Autodesk Fusion 360 part; units mm, degrees
(part 7 of 7)
  line L1008 (-19.5, -38.2) -> (-19.5, -32.2)
  line L1009 (-19.5, -32.2) -> (-19.5, -35.3676)
  circle A467 centre (-16.25, -62.1) radius 2.5
  circle A468 centre (-16.25, -62.1) radius 2.5
  line L1010 (34.2, 32.4) -> (59.7, 32.4)
  line L1011 (59.7, 32.4) -> (34.2, 32.4)
  line L1012 (95.9, -24.9) -> (101.9, -24.9)
  line L1013 (101.9, -24.9) -> (95.9, -24.9)
  line L1014 (-6.9778, -6.9) -> (-2, -6.9)
  line L1015 (-2, -6.9) -> (-2, -1.9)
  line L1016 (-2, -1.9) -> (-6.9716, -1.9)
  line L1017 (-6.9716, -1.9) -> (-6.9778, -6.9)
  line L1018 (46.45, -80.6) -> (45.65, -80.6)
  line L1019 (45.65, -80.6) -> (46.45, -80.6)
  line L1020 (107.65, -38.95) -> (107.65, -43.95)
  line L1021 (107.65, -43.95) -> (107.65, -38.95)
  line L1022 (-19.5, -44.7) -> (-19.5, -47.5324)
  line L1023 (-19.5, -47.5324) -> (-19.5, -50.7)
  line L1024 (-19.5, -50.7) -> (-19.5, -44.7)
  circle A469 centre (-16.25, -62.1) radius 0.4
  circle A470 centre (-16.25, -62.1) radius 0.4
  line L1025 (-2, -18.9) -> (-6.9926, -18.9)
  line L1026 (-6.9926, -18.9) -> (-2, -18.9)
  arc A471 (64.7, 8) -> (66.7, 10) centre (64.7, 10) ccw
  arc A472 (64.7, 8) -> (66.7, 10) centre (64.7, 10) ccw
  line L1027 (64.7, 8) -> (29.2, 8)
  line L1028 (29.2, 8) -> (64.7, 8)
  line L1029 (59.7, 32.4) -> (59.7, 30.4)
  line L1030 (59.7, 30.4) -> (59.7, 32.4)
  line L1031 (-6.9926, -18.9) -> (-6.9864, -13.9)
  line L1032 (-6.9864, -13.9) -> (-6.9926, -18.9)
  line L1033 (-19.5, -38.2) -> (-19.5, -35.3676)
  arc A473 (-19.5, -35.3676) -> (-22.3324, -38.2) centre (-16.25, -41.45) ccw
  line L1034 (-22.3324, -38.2) -> (-19.5, -38.2)
  line L1035 (59.7, 30.4) -> (66.7, 30.4)
  line L1036 (66.7, 30.4) -> (59.7, 30.4)
  line L1037 (107.2148, -43.61) -> (107.185, -39.2283)
  arc A474 (107.185, -39.2283) -> (98.0852, -39.29) centre (102.65, -41.45) ccw
  line L1038 (98.0852, -39.29) -> (98.115, -43.6717)
  arc A475 (98.115, -43.6717) -> (105.2701, -45.7671) centre (102.65, -41.45) ccw
  line L1039 (105.2701, -45.7671) -> (105.6552, -46.1523)
  line L1040 (105.6552, -46.1523) -> (107.3523, -44.4552)
  line L1041 (107.3523, -44.4552) -> (106.9671, -44.0701)
  arc A476 (106.9671, -44.0701) -> (107.2148, -43.61) centre (102.65, -41.45) ccw
  circle A477 centre (102.65, -41.45) radius 3.85
  line L1042 (-21.2106, -67.0687) -> (-21.5816, -73.1909)
  line L1043 (-21.5816, -73.1909) -> (-21.2106, -67.0687)
  line L1044 (101.9, -25.9) -> (95.9, -25.9)
  line L1045 (95.9, -25.9) -> (101.9, -25.9)
  line L1046 (101.9, -24.9) -> (101.9, -25.9)
  line L1047 (101.9, -25.9) -> (101.9, -24.9)
  arc A478 (-22.3324, -44.7) -> (-19.5, -47.5324) centre (-16.25, -41.45) ccw
  arc A479 (-22.3324, -44.7) -> (-19.5, -47.5324) centre (-16.25, -41.45) ccw
  line L1048 (-19.5, -44.7) -> (-22.3324, -44.7)
  arc A480 (-22.3324, -44.7) -> (-19.5, -47.5324) centre (-16.25, -41.45) ccw
  line L1049 (-19.5, -47.5324) -> (-19.5, -44.7)
  line L1050 (45.65, -79.6) -> (46.45, -79.6)
  line L1051 (46.45, -79.6) -> (45.65, -79.6)
  circle A481 centre (102.65, -41.45) radius 3.85
  circle A482 centre (102.65, -41.45) radius 3.85
  line L1052 (-7.5, -83.1) -> (-12.5, -83.1)
  line L1053 (-12.5, -83.1) -> (-7.5, -83.1)
  line L1054 (114.8523, -45.9448) -> (113.1552, -44.2477)
  line L1055 (113.1552, -44.2477) -> (114.8523, -45.9448)
  line L1056 (-12.5, -78.1) -> (-7.5, -83.1)
  line L1057 (-7.5, -83.1) -> (-12.5, -78.1)
  line L1058 (-7, 4.1) -> (-7, 2)
  line L1059 (-7, 2) -> (-7, 1.6)
  line L1060 (-7, 1.6) -> (-7, 4.1)
  line L1061 (48.25, -80.6) -> (47.45, -80.6)
  line L1062 (47.45, -80.6) -> (48.25, -80.6)
  line L1063 (114.4671, -46.3299) -> (114.8523, -45.9448)
  line L1064 (114.8523, -45.9448) -> (114.4671, -46.3299)
  line L1065 (-25.5, -38.2) -> (-25.5, -44.7)
  line L1066 (-25.5, -44.7) -> (-25.5, -38.2)
  line L1067 (-4.5, 4.1) -> (-7, 4.1)
  line L1068 (-7, 4.1) -> (-4.5, 4.1)
  line L1069 (112.7701, -44.6329) -> (113.1552, -44.2477)
  line L1070 (113.1552, -44.2477) -> (112.7701, -44.6329)
  line L1071 (-15.3557, -72.8958) -> (-20.5769, -73.1432)
  line L1072 (-20.5769, -73.1432) -> (-15.3557, -72.8958)
  arc A483 (-20.2671, -68.0326) -> (-15.3557, -72.8958) centre (-12.5, -65.1) ccw
  arc A484 (-20.2671, -68.0326) -> (-15.3557, -72.8958) centre (-12.5, -65.1) ccw
  arc A485 (48.25, -80.6) -> (48.25, -79.6) centre (48.25, -80.1) ccw
  arc A486 (48.25, -80.6) -> (48.25, -79.6) centre (48.25, -80.1) ccw
  line L1073 (-22.3324, -44.7) -> (-19.5, -44.7)
  line L1074 (-19.5, -44.7) -> (-25.5, -44.7)
  line L1075 (-25.5, -44.7) -> (-22.3324, -44.7)
  circle A487 centre (-4.5, 1.6) radius 0.4
  circle A488 centre (-4.5, 1.6) radius 0.4
  line L1076 (-10.1676, -38.2) -> (-13, -38.2)
  line L1077 (-13, -38.2) -> (-7, -38.2)
  line L1078 (-7, -38.2) -> (-10.1676, -38.2)
  arc A489 (-6.9678, 1.2) -> (-4.5, -0.9) centre (-4.5, 1.6) ccw
  arc A490 (-7, 1.6) -> (-4.5, -0.9) centre (-4.5, 1.6) ccw
  arc A491 (-7, 1.6) -> (-6.9678, 1.2) centre (-4.5, 1.6) ccw
  arc A492 (47.45, -79.6) -> (46.45, -79.6) centre (46.95, -79.6) ccw
  line L1079 (47.45, -79.6) -> (48.25, -79.6)
  arc A493 (48.25, -80.6) -> (48.25, -79.6) centre (48.25, -80.1) ccw
  line L1080 (48.25, -80.6) -> (47.45, -80.6)
  arc A494 (46.45, -80.6) -> (47.45, -80.6) centre (46.95, -80.6) ccw
  line L1081 (46.45, -80.6) -> (45.65, -80.6)
  arc A495 (45.65, -79.6) -> (45.65, -80.6) centre (45.65, -80.1) ccw
  line L1082 (45.65, -79.6) -> (46.45, -79.6)
  circle A496 centre (46.95, -80.1) radius 2.95
  circle A497 centre (-4.5, 1.6) radius 0.4
  line L1083 (113.1, -39.2591) -> (113.1, -43.6409)
  line L1084 (113.1, -43.6409) -> (113.1, -39.2591)
  line L1085 (122.2, -43.6409) -> (122.2, -39.2591)
  line L1086 (122.2, -39.2591) -> (122.2, -43.6409)
  line L1087 (-4.5, -0.9) -> (-2, -0.9)
  line L1088 (-2, -0.9) -> (-4.5, -0.9)
  line L1089 (13.4164, 23.7) -> (10.7819, 23.7)
  line L1090 (10.7819, 23.7) -> (27.2, 23.7)
  line L1091 (27.2, 23.7) -> (13.4164, 23.7)
  line L1092 (-6.5, -83.1) -> (-12.5, -77.1)
  line L1093 (-12.5, -77.1) -> (-6.5, -83.1)
  arc A498 (-20.617, -81.166) -> (-13.5, -83.0722) centre (-12.5, -65.1) ccw
  arc A499 (-20.617, -81.166) -> (-13.5, -83.0722) centre (-12.5, -65.1) ccw
  arc A500 (112.3409, -38.5) -> (112.3409, -29.4) centre (110.15, -33.95) ccw
  arc A501 (112.3409, -38.5) -> (112.3409, -29.4) centre (110.15, -33.95) ccw
  line L1094 (107.9591, -38.5) -> (112.3409, -38.5)
  line L1095 (112.3409, -38.5) -> (107.9591, -38.5)
  line L1096 (13.4164, 15.7) -> (27.2, 15.7)
  line L1097 (27.2, 15.7) -> (10.7819, 15.7)
  line L1098 (10.7819, 15.7) -> (13.4164, 15.7)
  line L1099 (122.2, -43.6409) -> (122.2, -39.2591)
  arc A502 (122.2, -39.2591) -> (115.0299, -37.1329) centre (117.65, -41.45) ccw
  line L1100 (115.0299, -37.1329) -> (114.6448, -36.7477)
  line L1101 (114.6448, -36.7477) -> (112.9477, -38.4448)
  line L1102 (112.9477, -38.4448) -> (113.3329, -38.8299)
  arc A503 (113.3329, -38.8299) -> (113.1, -39.2591) centre (117.65, -41.45) ccw
  line L1103 (113.1, -39.2591) -> (113.1, -43.6409)
  arc A504 (113.1, -43.6409) -> (122.2, -43.6409) centre (117.65, -41.45) ccw
  circle A505 centre (117.65, -41.45) radius 3.85
  line L1104 (0, 4.1) -> (-2, 4.1)
  line L1105 (-2, 4.1) -> (-4.5, 4.1)
  line L1106 (-4.5, 4.1) -> (0, 4.1)
  line L1107 (-13, -32.2) -> (-19.5, -32.2)
  line L1108 (-19.5, -32.2) -> (-13, -32.2)
  line L1109 (-27.8571, -74.4894) -> (-21.6425, -74.1949)
  line L1110 (-21.6425, -74.1949) -> (-27.8571, -74.4894)
  line L1111 (47.45, -79.6) -> (48.25, -79.6)
  line L1112 (48.25, -79.6) -> (47.45, -79.6)
  line L1113 (-13.5, -74.049) -> (-13.5, -83.0722)
  line L1114 (-13.5, -83.0722) -> (-13.5, -74.049)
  line L1115 (-19.5, -50.7) -> (-13, -50.7)
  line L1116 (-13, -50.7) -> (-19.5, -50.7)
  line L1117 (-23, 22.8505) -> (-23, 4.0495)
  line L1118 (-23, 4.0495) -> (-23, 22.8505)
  arc A506 (-27.8571, -74.4894) -> (-22.0173, -80.3781) centre (-12.5, -65.1) ccw
  line L1119 (-22.0173, -80.3781) -> (-21.6425, -74.1949)
  line L1120 (-21.6425, -74.1949) -> (-27.8571, -74.4894)
  line L1121 (-21.0008, -80.1355) -> (-14.7326, -73.8674)
  line L1122 (-14.7326, -73.8674) -> (-20.6378, -74.1472)
  line L1123 (-20.6378, -74.1472) -> (-21.0008, -80.1355)
  line L1124 (-8.1652, 16.7) -> (8.1652, 16.7)
  line L1125 (8.1652, 16.7) -> (-8.1652, 16.7)
  line L1126 (-20.5769, -73.1432) -> (-15.3557, -72.8958)
  arc A507 (-20.2671, -68.0326) -> (-15.3557, -72.8958) centre (-12.5, -65.1) ccw
  line L1127 (-20.2671, -68.0326) -> (-20.5769, -73.1432)
  line L1128 (118.9, -24.9) -> (119.9, -24.9)
  line L1129 (119.9, -24.9) -> (118.9, -24.9)
  line L1130 (112.3409, -29.4) -> (107.9591, -29.4)
  line L1131 (107.9591, -29.4) -> (112.3409, -29.4)
  line L1132 (112.3409, -44.4) -> (107.9591, -44.4)
  line L1133 (107.9591, -44.4) -> (112.3409, -44.4)
  arc A508 (-8.1652, 16.7) -> (-8.1652, 14.7) centre (-8.1652, 15.7) ccw
  arc A509 (-8.1652, 16.7) -> (-8.1652, 14.7) centre (-8.1652, 15.7) ccw
  line L1134 (-20.5769, -73.1432) -> (-20.2671, -68.0326)
  line L1135 (-20.2671, -68.0326) -> (-20.5769, -73.1432)
  line L1136 (-22, 4.0495) -> (-22, 22.8505)
  line L1137 (-22, 22.8505) -> (-22, 4.0495)
  line L1138 (-12.5, -78.1) -> (-12.5, -83.1)
  line L1139 (-12.5, -83.1) -> (-7.5, -83.1)
  line L1140 (-7.5, -83.1) -> (-12.5, -78.1)
  arc A510 (113.1, -43.6409) -> (122.2, -43.6409) centre (117.65, -41.45) ccw
  arc A511 (113.1, -43.6409) -> (122.2, -43.6409) centre (117.65, -41.45) ccw
  line L1141 (-13, -47.5324) -> (-13, -44.7)
  line L1142 (-13, -44.7) -> (-13, -50.7)
  line L1143 (-13, -50.7) -> (-13, -47.5324)
  line L1144 (-20.6378, -74.1472) -> (-14.7326, -73.8674)
  line L1145 (-14.7326, -73.8674) -> (-20.6378, -74.1472)
  line L1146 (-21.0008, -80.1355) -> (-20.6378, -74.1472)
  line L1147 (-20.6378, -74.1472) -> (-21.0008, -80.1355)
  line L1148 (-20.617, -81.166) -> (-13.5, -74.049)
  line L1149 (-13.5, -74.049) -> (-20.617, -81.166)
  arc A512 (112.7701, -44.6329) -> (112.3409, -44.4) centre (110.15, -48.95) ccw
  arc A513 (112.7701, -44.6329) -> (112.3409, -44.4) centre (110.15, -48.95) ccw
  line L1150 (-14.7326, -73.8674) -> (-21.0008, -80.1355)
  line L1151 (-21.0008, -80.1355) -> (-14.7326, -73.8674)
  arc A514 (-27.8571, -74.4894) -> (-22.0173, -80.3781) centre (-12.5, -65.1) ccw
  arc A515 (-27.8571, -74.4894) -> (-22.0173, -80.3781) centre (-12.5, -65.1) ccw
  arc A516 (122.2, -39.2591) -> (115.0299, -37.1329) centre (117.65, -41.45) ccw
  arc A517 (122.2, -39.2591) -> (115.0299, -37.1329) centre (117.65, -41.45) ccw
  line L1152 (-21.6425, -74.1949) -> (-22.0173, -80.3781)
  line L1153 (-22.0173, -80.3781) -> (-21.6425, -74.1949)
  line L1154 (115.0299, -37.1329) -> (114.6448, -36.7477)
  line L1155 (114.6448, -36.7477) -> (115.0299, -37.1329)
  line L1156 (113.3329, -38.8299) -> (112.9477, -38.4448)
  line L1157 (112.9477, -38.4448) -> (113.3329, -38.8299)
  arc A518 (113.3329, -38.8299) -> (113.1, -39.2591) centre (117.65, -41.45) ccw
  arc A519 (113.3329, -38.8299) -> (113.1, -39.2591) centre (117.65, -41.45) ccw
  arc A520 (47.45, -79.6) -> (46.45, -79.6) centre (46.95, -79.6) ccw
  arc A521 (47.45, -79.6) -> (46.45, -79.6) centre (46.95, -79.6) ccw
  arc A522 (0, 5.7) -> (8.6603, 8.7) centre (0, 19.7) ccw
  line L1158 (0, 5.7) -> (0, 4.1)
  line L1159 (0, 4.1) -> (27.2, 4.1)
  line L1160 (27.2, 4.1) -> (27.2, 8.7)
  line L1161 (27.2, 8.7) -> (8.6603, 8.7)
  circle A523 centre (46.95, -80.1) radius 2.95
  arc A524 (46.4092, -77.2) -> (47.4908, -77.2) centre (46.95, -80.1) ccw
  arc A525 (47.4908, -77.2) -> (46.4092, -77.2) centre (46.95, -80.1) ccw
  line L1162 (27.2, 30.4) -> (34.2, 30.4)
  line L1163 (34.2, 30.4) -> (27.2, 30.4)
  arc A526 (-19.8023, -65.1) -> (-12.5, -72.4023) centre (-12.5, -65.1) ccw
  arc A527 (-19.8023, -65.1) -> (-12.5, -72.4023) centre (-12.5, -65.1) ccw
  line L1164 (-23, 22.8505) -> (-23, 4.0495)
  arc A528 (-22, 4.0495) -> (-23, 4.0495) centre (-22.5, 1.6) ccw
  line L1165 (-22, 4.0495) -> (-22, 22.8505)
  arc A529 (-23, 22.8505) -> (-22, 22.8505) centre (-22.5, 25.3) ccw
  line L1166 (-12.5, -77.1) -> (-12.5, -72.4023)
  line L1167 (-12.5, -72.4023) -> (-12.5, -77.1)
  line L1168 (-12.5, -84.1) -> (-6.5, -84.1)
  line L1169 (-6.5, -84.1) -> (-12.5, -84.1)
  line L1170 (27.2, 15.7) -> (13.4164, 15.7)
  arc A530 (8.6603, 8.7) -> (13.4164, 15.7) centre (0, 19.7) ccw
  line L1171 (8.6603, 8.7) -> (27.2, 8.7)
  line L1172 (27.2, 8.7) -> (27.2, 15.7)
  arc A531 (8.1652, 14.7) -> (8.1652, 16.7) centre (8.1652, 15.7) ccw
  arc A532 (8.1652, 14.7) -> (8.1652, 16.7) centre (8.1652, 15.7) ccw
  arc A533 (-20.617, -81.166) -> (-13.5, -83.0722) centre (-12.5, -65.1) ccw
  line L1173 (-13.5, -83.0722) -> (-13.5, -74.049)
  line L1174 (-13.5, -74.049) -> (-20.617, -81.166)
  line L1175 (-31.5, 4.1) -> (-31.5, 25.3)
  line L1176 (-31.5, 25.3) -> (-31.5, 4.1)
  line L1177 (124.4, -7.9) -> (124.4, -12.9)
  line L1178 (124.4, -12.9) -> (124.4, -7.9)
  line L1179 (119.9, -0.9) -> (119.9, 4.1)
  line L1180 (119.9, 4.1) -> (119.9, -0.9)
  line L1181 (98.4, 4.1) -> (95.9, 4.1)
  line L1182 (95.9, 4.1) -> (98.4, 4.1)
  line L1183 (124.4, -0.9) -> (119.9, -0.9)
  line L1184 (119.9, -0.9) -> (124.4, -0.9)
  arc A534 (102.0652, 14.7) -> (102.0652, 16.7) centre (102.0652, 15.7) ccw
  arc A535 (102.0652, 14.7) -> (102.0652, 16.7) centre (102.0652, 15.7) ccw
  line L1185 (85.7348, 24.7) -> (102.0652, 24.7)
  line L1186 (102.0652, 24.7) -> (85.7348, 24.7)
  line L1187 (102.9, 18.7) -> (84.9, 18.7)
  line L1188 (84.9, 18.7) -> (102.9, 18.7)
  line L1189 (95.9, 4.1) -> (93.9, 4.1)
  line L1190 (93.9, 4.1) -> (95.9, 4.1)
  line L1191 (118.9, 1.6) -> (118.9, 4.1)
  line L1192 (118.9, 4.1) -> (118.9, 1.6)
  arc A536 (83.1181, 15.7) -> (83.1181, 23.7) centre (93.9, 19.7) ccw
  arc A537 (83.1181, 15.7) -> (83.1181, 23.7) centre (93.9, 19.7) ccw
  line L1193 (98.9, 10.7) -> (88.9, 10.7)
  line L1194 (88.9, 10.7) -> (98.9, 10.7)
  line L1195 (107.9, -0.9) -> (107.9, 1.2)
  line L1196 (107.9, 1.2) -> (107.9, -0.9)
  line L1197 (116.9, 4.0495) -> (116.9, 22.8505)
  arc A538 (115.9, 22.8505) -> (116.9, 22.8505) centre (116.4, 25.3) ccw
  line L1198 (115.9, 22.8505) -> (115.9, 4.0495)
  arc A539 (116.9, 4.0495) -> (115.9, 4.0495) centre (116.4, 1.6) ccw
  circle A540 centre (116.4, 25.3) radius 2.5
  arc A541 (116.9, 22.8505) -> (115.9, 22.8505) centre (116.4, 25.3) ccw
  arc A542 (115.9, 22.8505) -> (116.9, 22.8505) centre (116.4, 25.3) ccw
  line L1199 (107.9, 1.2) -> (107.9, -0.9)
  line L1200 (107.9, -0.9) -> (112.9, -0.9)
  line L1201 (112.9, -0.9) -> (112.9, 1.2)
  line L1202 (112.9, 1.2) -> (107.9, 1.2)
  line L1203 (116.4, -0.9) -> (113.9, -0.9)
  line L1204 (113.9, -0.9) -> (116.4, -0.9)
  arc A543 (102.0652, 22.7) -> (102.0652, 24.7) centre (102.0652, 23.7) ccw
  arc A544 (102.0652, 22.7) -> (102.0652, 24.7) centre (102.0652, 23.7) ccw
  line L1205 (113.9, 1.2) -> (113.9, -0.9)
  line L1206 (113.9, -0.9) -> (116.4, -0.9)
  arc A545 (113.9322, 1.2) -> (116.4, -0.9) centre (116.4, 1.6) ccw
  line L1207 (113.9322, 1.2) -> (113.9, 1.2)
  line L1208 (124.4, -0.9) -> (124.4, 4.1)
  line L1209 (124.4, 4.1) -> (119.9, 4.1)
  line L1210 (119.9, 4.1) -> (119.9, -0.9)
  line L1211 (119.9, -0.9) -> (124.4, -0.9)
  circle A546 centre (116.4, 25.3) radius 0.4
  circle A547 centre (116.4, 25.3) radius 0.4
  line L1212 (88.8996, 12.7) -> (98.8996, 12.7)
  line L1213 (98.8996, 12.7) -> (88.8996, 12.7)
  circle A548 centre (110.2363, -20.8316) radius 0.4
  circle A549 centre (110.2363, -20.8316) radius 0.4
  line L1214 (118.9, -24.9) -> (118.9, -25.9)
  line L1215 (118.9, -25.9) -> (124.4, -25.9)
  line L1216 (124.4, -25.9) -> (124.4, -24.9)
  line L1217 (124.4, -24.9) -> (124.4, -19.9)
  line L1218 (124.4, -19.9) -> (119.9, -19.9)
  line L1219 (119.9, -19.9) -> (119.9, -24.9)
  line L1220 (119.9, -24.9) -> (118.9, -24.9)
  arc A550 (116.4, 2) -> (116.3992, 1.2) centre (116.4, 1.6) ccw
  arc A551 (116.3992, 1.2) -> (116.4, 2) centre (116.4, 1.6) ccw
  line L1221 (119.9, -12.9) -> (119.9, -7.9)
  line L1222 (119.9, -7.9) -> (119.9, -12.9)
  line L1223 (98.9004, 26.7) -> (88.8996, 26.7)
  line L1224 (88.8996, 26.7) -> (98.9004, 26.7)
  arc A552 (98.9004, 26.7) -> (98.9, 28.7) centre (98.9, 27.7) ccw
  arc A553 (98.9004, 26.7) -> (98.9, 28.7) centre (98.9, 27.7) ccw
  line L1225 (119.9, -19.9) -> (124.4, -19.9)
  line L1226 (124.4, -19.9) -> (119.9, -19.9)
  line L1227 (116.4, -0.9) -> (118.9, -0.9)
  line L1228 (118.9, -0.9) -> (116.4, -0.9)
  line L1229 (124.4, 4.1) -> (124.4, -0.9)
  line L1230 (124.4, -0.9) -> (124.4, 4.1)
  line L1231 (113.9, -0.9) -> (113.9, 1.2)
  line L1232 (113.9, 1.2) -> (113.9, -0.9)
  line L1233 (100.8678, 1.2) -> (100.8704, -0.9)
  line L1234 (100.8704, -0.9) -> (100.8678, 1.2)
  line L1235 (119.9, -7.9) -> (124.4, -7.9)
  line L1236 (124.4, -7.9) -> (119.9, -7.9)
  line L1237 (116.4, -0.9) -> (118.9, -0.9)
  line L1238 (118.9, -0.9) -> (118.9, 1.6)
  arc A554 (116.4, -0.9) -> (118.9, 1.6) centre (116.4, 1.6) ccw
  line L1239 (100.9, 4.1) -> (98.4, 4.1)
  line L1240 (98.4, 4.1) -> (100.9, 4.1)
  line L1241 (98.4, -0.9) -> (100.8704, -0.9)
  line L1242 (100.8704, -0.9) -> (100.8678, 1.2)
  arc A555 (98.4, -0.9) -> (100.8678, 1.2) centre (98.4, 1.6) ccw
  line L1243 (118.9, 1.6) -> (118.9, -0.9)
  line L1244 (118.9, -0.9) -> (118.9, 1.6)
  arc A556 (98.9, 10.7) -> (98.8996, 12.7) centre (98.9, 11.7) ccw
  arc A557 (98.9, 10.7) -> (98.8996, 12.7) centre (98.9, 11.7) ccw
  circle A558 centre (116.4, 25.3) radius 0.4
  line L1245 (119.9, -7.9) -> (119.9, -12.9)
  line L1246 (119.9, -12.9) -> (124.4, -12.9)
  line L1247 (124.4, -12.9) -> (124.4, -7.9)
  line L1248 (124.4, -7.9) -> (119.9, -7.9)
  line L1249 (112.9, -0.9) -> (107.9, -0.9)
  line L1250 (107.9, -0.9) -> (112.9, -0.9)
  line L1251 (85.7348, 16.7) -> (102.0652, 16.7)
  line L1252 (102.0652, 16.7) -> (85.7348, 16.7)
  circle A559 centre (110.2363, -20.8316) radius 0.4
  line L1253 (102.0652, 14.7) -> (85.7348, 14.7)
  line L1254 (85.7348, 14.7) -> (102.0652, 14.7)
  line L1255 (98.4, -0.9) -> (100.8704, -0.9)
  line L1256 (100.8704, -0.9) -> (98.4, -0.9)
  arc A560 (102.9, 18.7) -> (102.9, 20.7) centre (102.9, 19.7) ccw
  arc A561 (102.9, 18.7) -> (102.9, 20.7) centre (102.9, 19.7) ccw
  line L1257 (112.9, 1.2) -> (112.9, -0.9)
  line L1258 (112.9, -0.9) -> (112.9, 1.2)
  line L1259 (102.0652, 22.7) -> (85.7348, 22.7)
  line L1260 (85.7348, 22.7) -> (102.0652, 22.7)
  line L1261 (124.4, -12.9) -> (119.9, -12.9)
  line L1262 (119.9, -12.9) -> (124.4, -12.9)
  line L1263 (88.9, 28.7) -> (98.9, 28.7)
  line L1264 (98.9, 28.7) -> (88.9, 28.7)
  line L1265 (124.4, -19.9) -> (124.4, -24.9)
  line L1266 (124.4, -24.9) -> (124.4, -19.9)
  line L1267 (84.9, 20.7) -> (102.9, 20.7)
  line L1268 (102.9, 20.7) -> (84.9, 20.7)
  line L1269 (119.9, -24.9) -> (119.9, -19.9)
  line L1270 (119.9, -19.9) -> (119.9, -24.9)
  spline S23 degree 3 poles (126.7177, -15.6596) (127.0784, -14.2999) (127.2562, -12.8809) (127.2612, -10.0454) (127.0837, -8.6064) (126.7183, -7.2283) knots 0 0 0 0 0.422012 0.422012 0.849727 0.849727 0.849727 0.849727
  ellipse E6 centre (131.4, -18.1364) end of major axis (131.4, -11.0757) minor radius 5 (126.7177, -15.6596) -> (126.4, -18.1364) ccw
  line L1271 (126.4, -18.1364) -> (126.4, -4.7455)
  ellipse E7 centre (131.4, -4.7455) end of major axis (131.4, -11.8166) minor radius 5 (126.4, -4.7455) -> (126.7183, -7.2283) ccw
  line L1272 (96.4, 35.3) -> (96.4, 34.3)
  line L1273 (96.4, 34.3) -> (96.4, 35.3)
  point P0 (-25, 4.1)
  point P1 (116.4, -0.9)
  point P2 (118.9, 1.6)
  point P3 (98.4, -0.9)
  point P4 (-25, 1.6)
  point P5 (-20.0322, 1.2)
  point P6 (-22.5, 35.3)
  point P7 (-6.9678, 1.2)
  point P8 (95.9, 4.1)
  point P9 (118.9, 1.6)
sketch "ExportDXFOnlyPCB" plane through (0, 0, 2.4) normal (0, 0, -1) x (1, 0, 0)
  line L0 (24.5, -81.15) -> (24.5, -83.65)
  line L1 (24.5, -83.65) -> (95.9, -83.65)
  line L2 (95.9, -83.65) -> (95.9, -3.65)
  line L3 (95.9, -3.65) -> (100.9, -3.65)
  line L4 (100.9, -3.65) -> (100.9, 4.1)
  line L5 (100.9, 4.1) -> (-7, 4.1)
  line L6 (-7, 4.1) -> (-7, -3.65)
  line L7 (-7, -3.65) -> (-2, -3.65)
  line L8 (-2, -3.65) -> (-2, -83.65)
  line L9 (-2, -83.65) -> (16.5, -83.65)
  line L10 (16.5, -83.65) -> (16.5, -77.2)
  line L11 (16.5, -77.2) -> (24.5, -77.2)
  line L12 (24.5, -77.2) -> (24.5, -81.15)
  circle A0 centre (84.4, -5) radius 2.5
  circle A1 centre (98.4, 1.6) radius 1
  circle A2 centre (73.4, -81.15) radius 1
  circle A3 centre (-4.5, 1.6) radius 1
  circle A4 centre (80.15, -44.4) radius 2.5
  circle A5 centre (8, -81.15) radius 1
  circle A6 centre (10.06, -44.3) radius 2.5
sketch "ExportDXFDSPCB" plane through (0, 0, -13.7) normal (0, 0, -1) x (1, 0, 0)
  circle A0 centre (84.4, -5) radius 1.5
  circle A1 centre (-3.4, 0) radius 1.5
  circle A2 centre (10.06, -44.3) radius 2
  circle A3 centre (-14.9, 17.5) radius 2
  circle A4 centre (80.15, -44.4) radius 2
  circle A5 centre (103.9, 17.5) radius 2
  line L0 (77.6, 34.7) -> (16.3, 34.7)
  line L1 (16.3, 34.7) -> (16.3, 28.2)
  line L2 (16.3, 28.2) -> (18.6, 28.2)
  line L3 (18.6, 28.2) -> (18.6, 10.2)
  line L4 (18.6, 10.2) -> (16.3, 10.2)
  line L5 (16.3, 10.2) -> (16.3, 21)
  line L6 (16.3, 21) -> (-18.4, 21)
  line L7 (-18.4, 21) -> (-18.4, -42.54)
  line L8 (-18.4, -42.54) -> (6.28, -42.54)
  line L9 (6.28, -42.54) -> (6.28, -47.8)
  line L10 (6.28, -47.8) -> (69.9, -47.8)
  line L11 (69.9, -47.8) -> (69.9, -42)
  line L12 (69.9, -42) -> (76.4, -42)
  line L13 (76.4, -42) -> (76.4, -47.8)
  line L14 (76.4, -47.8) -> (83.9, -47.8)
  line L15 (83.9, -47.8) -> (83.9, -41.2)
  line L16 (83.9, -41.2) -> (95.4, -41.2)
  line L17 (95.4, -41.2) -> (95.4, -47.8)
  line L18 (95.4, -47.8) -> (107.4, -47.8)
  line L19 (107.4, -47.8) -> (107.4, 21)
  line L20 (107.4, 21) -> (77.6, 21)
  line L21 (77.6, 21) -> (77.6, 10.2)
  line L22 (77.6, 10.2) -> (75.3, 10.2)
  line L23 (75.3, 10.2) -> (75.3, 28.2)
  line L24 (75.3, 28.2) -> (77.6, 28.2)
  line L25 (77.6, 28.2) -> (77.6, 34.7)
sketch "Sketch108" plane through (0, 0, 13.6) normal (0, 0, -1) x (1, 0, 0)
  line L0 (126.4, -65.1) -> (125.4, -65.1)
  line L1 (125.4, -65.1) -> (125.4, 4.1)
  line L2 (125.4, 4.1) -> (124.4, 4.1)
  line L3 (124.4, 4.1) -> (124.4, -0.9)
  line L4 (124.4, -0.9) -> (119.9, -0.9)
  line L5 (119.9, -0.9) -> (119.9, 4.1)
  line L6 (119.9, 4.1) -> (118.9, 4.1)
  line L7 (118.9, 4.1) -> (118.9, 1.6)
  line L8 (118.9, 1.6) -> (118.9, -0.9)
  line L9 (118.9, -0.9) -> (116.4, -0.9)
  line L10 (116.4, -0.9) -> (113.9, -0.9)
  line L11 (113.9, -0.9) -> (113.9, 1.2)
  line L12 (113.9, 1.2) -> (112.9, 1.2)
  line L13 (112.9, 1.2) -> (112.9, -0.9)
  line L14 (112.9, -0.9) -> (107.9, -0.9)
  line L15 (107.9, -0.9) -> (107.9, 1.2)
  line L16 (107.9, 1.2) -> (100.8678, 1.2)
  line L17 (100.8678, 1.2) -> (100.8704, -0.9)
  line L18 (100.8704, -0.9) -> (98.4, -0.9)
  line L19 (98.4, -0.9) -> (95.9, -0.9)
  line L20 (95.9, -0.9) -> (95.9, -24.9)
  line L21 (95.9, -24.9) -> (101.9, -24.9)
  line L22 (101.9, -24.9) -> (101.9, -25.9)
  line L23 (101.9, -25.9) -> (95.9, -25.9)
  line L24 (95.9, -25.9) -> (95.9, -77.2)
  line L25 (95.9, -77.2) -> (75.9, -77.2)
  line L26 (75.9, -77.2) -> (75.9, -85.1)
  line L27 (75.9, -85.1) -> (106.4, -85.1)
  arc A0 (106.4, -85.1) -> (126.4, -65.1) centre (106.4, -65.1) ccw
  line L28 (118.9, -24.9) -> (119.9, -24.9)
  line L29 (119.9, -24.9) -> (119.9, -19.9)
  line L30 (119.9, -19.9) -> (124.4, -19.9)
  line L31 (124.4, -19.9) -> (124.4, -24.9)
  line L32 (124.4, -24.9) -> (124.4, -25.9)
  line L33 (124.4, -25.9) -> (118.9, -25.9)
  line L34 (118.9, -25.9) -> (118.9, -24.9)
  line L35 (119.9, -7.9) -> (124.4, -7.9)
  line L36 (124.4, -7.9) -> (124.4, -12.9)
  line L37 (124.4, -12.9) -> (119.9, -12.9)
  line L38 (119.9, -12.9) -> (119.9, -7.9)
  circle A1 centre (110.15, -62.1) radius 2.5
  circle A2 centre (110.2363, -20.8316) radius 2.5
  circle A3 centre (102.65, -41.45) radius 3.85
  circle A4 centre (110.15, -48.95) radius 3.85
  circle A5 centre (117.6453, -56.4453) radius 2.35
  circle A6 centre (110.15, -33.95) radius 3.85
  circle A7 centre (102.6547, -56.4453) radius 2.35
  circle A8 centre (117.65, -41.45) radius 3.85
  line L39 (112.3409, -38.5) -> (107.9591, -38.5)
  line L40 (107.9591, -53.5) -> (112.3364, -53.5)
  line L41 (98.0852, -39.29) -> (98.115, -43.6717)
  line L42 (102.65, -35.45) -> (104.15, -35.45)
  line L43 (104.15, -33.95) -> (104.15, -35.45)
  line L44 (117.65, -35.45) -> (116.15, -35.45)
  line L45 (116.15, -33.95) -> (116.15, -35.45)
  arc A9 (116.15, -33.95) -> (104.15, -33.95) centre (110.15, -33.95) ccw
  line L46 (104.15, -33.95) -> (104.15, -35.45)
  line L47 (117.65, -47.45) -> (116.15, -47.45)
  line L48 (116.15, -48.95) -> (116.15, -47.45)
  arc A10 (117.65, -47.45) -> (117.65, -35.45) centre (117.65, -41.45) ccw
  line L49 (104.15, -48.95) -> (104.15, -47.45)
  arc A11 (102.65, -35.45) -> (102.65, -47.45) centre (102.65, -41.45) ccw
  line L50 (102.65, -47.45) -> (104.15, -47.45)
  arc A12 (104.15, -48.95) -> (105.0008, -52.03) centre (110.15, -48.95) ccw
  arc A13 (105.0008, -52.03) -> (107.07, -54.0992) centre (102.6547, -56.4453) ccw
  arc A14 (107.07, -54.0992) -> (113.23, -54.0992) centre (110.15, -48.95) ccw
  arc A15 (115.2992, -52.03) -> (116.15, -48.95) centre (110.15, -48.95) ccw
  arc A16 (113.23, -54.0992) -> (115.2992, -52.03) centre (117.6453, -56.4453) ccw
  point P0 (107.65, -38.95)
  point P1 (112.65, -43.95)
  constraint concentric A7 A13
  constraint concentric A5 A16
  constraint concentric A3 A11
  constraint tangent L42 A11
  constraint tangent A11 L50
  constraint concentric A12 A14
  constraint concentric A14 A15
extrude "Extrude91" cut sketch "Sketch108" against normal blind 1 contours L42 L43 L44 L45 A9 L46 L47 L48 A10 L49 A11 L50 A12 A13 A14 A15 A16 bodies 3
hidden bodies 1
equation "d42 = ( 7.5 / 2 ) * 1 mm"
equation "d43 = ( 7.5 / 2 ) * 1 mm"
equation "d44 = ( 7.5 / 2 ) * 1 mm"
equation "d45 = ( 7.5 / 2 ) * 1 mm"
equation "d46 = ( 7.5 / 2 ) * 1 mm"
equation "d47 = ( 7.5 / 2 ) * 1 mm"
equation "d59 = ( 6.5 / 2 ) * 1 mm"
equation "d61 = ( 6.5 / 2 ) * 1 mm"
equation "d62 = ( 6.5 / 2 ) * 1 mm"
equation "d63 = ( 6.5 / 2 ) * 1 mm"
equation "d64 = ( 6.5 / 2 ) * 1 mm"
equation "d65 = ( 6.5 / 2 ) * 1 mm"
equation "d66 = ( 6.5 / 2 ) * 1 mm"
equation "d75 = 27.5 mm - 6 mm"
equation "d136 = ( 2.3 * 2 ) * 1 mm"
equation "d340 = ( 5.9 / 2 ) * 1 mm"
equation "d498 = 24 mm - 5.6 mm"
named bodies: "Screen", "PCB", "MAIN", "Ctrl-ABXY", "struct-up", "Little", "struct-down", "NewPCB"
